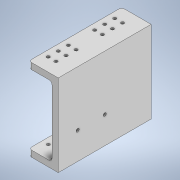
# Autodesk Inventor part: Part1
Saved by Autodesk Inventor 2020.3 (Build 243373000, 373)
## iProperties
Created: 2020-07-15
Part Number: Part1
Material: Generic
Document SubType Name: Modeling
Designer: mifer
Density: 1 g/cm^3
Appearance: Default
Author: mifer
## iProperties of the stored document _3DPrint.ipt
Created: 2020-07-15
Part Number: _3DPrint
Material: Generic
Document SubType Name: Modeling
Designer: mifer
Density: 1 g/cm^3
Appearance: Default
Author: mifer
Autodesk Inventor part; units mm, degrees
ref_plane "YZ Plane" through (0, 0, 0) normal (1, 0, 0) x (0, 1, 0)
ref_plane "XZ Plane" through (0, 0, 0) normal (0, 1, 0) x (-1, 0, 0)
sketch "Sketch1" plane through (0, 0, 0) normal (0, 1, 0) x (-1, 0, 0)
  line L0 (0, 0) -> (8, 0)
  line L1 (8, 0) -> (8, -120)
  line L2 (8, -120) -> (0, -120)
  line L3 (0, -120) -> (0, 0)
  line L4 (8, 0) -> (38, 0)
  line L5 (38, 0) -> (38, -120)
  line L6 (38, -120) -> (8, -120)
  line L7 (8, -120) -> (8, 0)
  circle A0 centre (20, -17) radius 2
  circle A1 centre (20, -30) radius 2
  circle A2 centre (20, -43) radius 2
  circle A3 centre (20, -77) radius 2
  circle A4 centre (20, -90) radius 2
  circle A5 centre (20, -103) radius 2
  circle A6 centre (30, -17) radius 2
  circle A7 centre (30, -30) radius 2
  circle A8 centre (30, -43) radius 2
  circle A9 centre (30, -77) radius 2
  circle A10 centre (30, -90) radius 2
  circle A11 centre (30, -103) radius 2
  dimension "d15" = 8
  dimension "d16" = 120
  dimension "d17" = 30
  constraints: 16 end point, 12 centre point, 4 parallel, 2 horizontal, 2 perpendicular
  measures "d15" distance of L1.end L2.end
  measures "d16" distance of L0.end L1.end
  measures "d17" distance of L5.end L6.end
extrude "Extrusion3" add sketch "Sketch1" along normal blind 98 contours L0 L1 L2 L3
extrude "Extrusion4" add sketch "Sketch1" along normal blind 8 contours L4 L5 L6 L1
sketch "Sketch2" plane through (0, 0, 0) normal (1, 0, 0) x (0, 0, -1)
  line L0 (0, 0) -> (120, 0) projected
  line L1 (120, 0) -> (120, 98) projected
  line L2 (0, 0) -> (0, 35)
  line L3 (0, 8) -> (0, 98) projected
  circle A0 centre (25, 35) radius 2
  circle A1 centre (60, 35) radius 2
  dimension "d53" = 4
  dimension "d54" = 4
  constraints: 2 centre point, 2 end point, 1 point on line
  measures "d53" diameter of A0
  measures "d54" diameter of A1
extrude "Extrusion5" cut sketch "Sketch2" against normal blind 10
ref_plane "Work Plane1" through (0, 98, 0) normal (0, -1, 0) x (1, 0, 0)
sketch "Sketch4" plane through (0, 98, 0) normal (0, -1, 0) x (1, 0, 0)
  line L0 (0, -120) -> (0, 0)
  line L1 (0, 0) -> (-8, 0)
  line L2 (-8, 0) -> (-8, -120)
  line L3 (-8, -120) -> (0, -120)
  line L4 (-8, 0) -> (-38, 0)
  line L5 (-38, 0) -> (-38, -120)
  line L6 (-38, -120) -> (-8, -120)
  line L7 (-8, -120) -> (-8, 0)
  circle A0 centre (-20, -17) radius 2
  circle A1 centre (-20, -30) radius 2
  circle A2 centre (-20, -43) radius 2
  circle A3 centre (-20, -77) radius 2
  circle A4 centre (-20, -90) radius 2
  circle A5 centre (-20, -103) radius 2
  circle A6 centre (-30, -77) radius 2
  circle A7 centre (-30, -90) radius 2
  circle A8 centre (-30, -103) radius 2
  circle A9 centre (-30, -43) radius 2
  circle A10 centre (-30, -30) radius 2
  circle A11 centre (-30, -17) radius 2
  point P0 (8, -120)
  constraints: 16 end point, 12 centre point
extrude "Extrusion6" add sketch "Sketch4" against normal blind 8
fillet "Fillet1" radius 4 6 edges at (-38, 102, 0) (-38, 102, -120) (-38, 4, -120) (-38, 4, 0) (-8, 98, -60) (-8, 8, -60)
body "Solid2"
